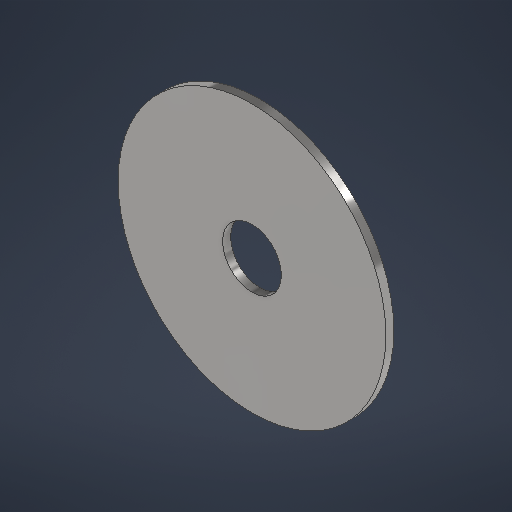
# Autodesk Inventor part: Friction Plate
Saved by Autodesk Inventor 2026.3 (Build 303398000, 398)
## iProperties
Created: 2026-07-28
Part Number: Friction Plate
Material: Generic
Document SubType Name: Sheet Metal
Designer: matot
Density: 1 g/cm^3
Sheet Metal Rule: Default_mm
Appearance: Default
Flat Pattern Width: 10 cm
Flat Pattern Length: 10 cm
Flat Pattern Area: 100 cm^2
Sheet Metal Width: 100.000 mm
Sheet Metal Length: 100.000 mm
Sheet Metal Area: 10000.000 mm^2
Author: matot
Autodesk Inventor part; units mm, degrees
ref_plane "YZ Plane" through (0, 0, 0) normal (1, 0, 0) x (0, 1, 0)
ref_plane "XZ Plane" through (0, 0, 0) normal (0, 1, 0) x (-1, 0, 0)
ref_plane "XY Plane" through (0, 0, 0) normal (0, 0, 1) x (1, 0, 0)
sketch "Sketch1" plane through (0, 0, 0) normal (0, 0, 1) x (1, 0, 0)
  circle A0 centre (0, 0) radius 50
  circle A1 centre (0, 0) radius 11
  dimension "d0" = 100
  dimension "d3" = 22
  constraints: 2 centre point, 2 coincident
  measures "d0" diameter of A0
  measures "d3" diameter of A1
extrude "Extrusion1" add sketch "Sketch1" along normal blind 3 contours A0 | A1
sketch "Sketch2" plane through (0, 0, 3) normal (0, 0, 1) x (1, 0, 0)
  circle A0 centre (0, 0) radius 11
  dimension "d4" = 22
  constraints: 1 centre point, 1 coincident
  measures "d4" diameter of A0
extrude "Extrusion2" cut sketch "Sketch2" against normal through all
sketch "Sketch3" plane through (0, 0, 3) normal (0, 0, 1) x (1, 0, 0)
  point P0 (0, 0)
  point P1 (-23.6, 25.4)
  point P2 (23.5, -25.5)
  dimension "d7" = 25.4
  dimension "d8" = 23.6
  dimension "d9" = 25.5
  dimension "d10" = 23.5
  measures "d7" vertical distance of point (0, 0) point (-23.6, 25.4)
  measures "d8" horizontal distance of point (0, 0) point (-23.6, 25.4)
  measures "d9" vertical distance of point (0, 0) point (23.5, -25.5)
  measures "d10" horizontal distance of point (0, 0) point (23.5, -25.5)
hole "Hole1" [suppressed]
equation "\"d16\" = Thickness"
equation "\"BendRadius\" = Thickness"
equation "\"BendReliefWidth\" = Thickness"
equation "\"BendReliefDepth\" = 0.5 * Thickness"
equation "\"CornerReliefSize\" = 4 * Thickness"
equation "\"MinimumRemnant\" = 2 * Thickness"
equation "\"TransitionRadius\" = BendRadius"
equation "\"JacobiRadiusSize\" = BendRadius"
equation "\"GapSize\" = Thickness"
equation "\"Thickness\" = 0.5"
body "Solid1"
